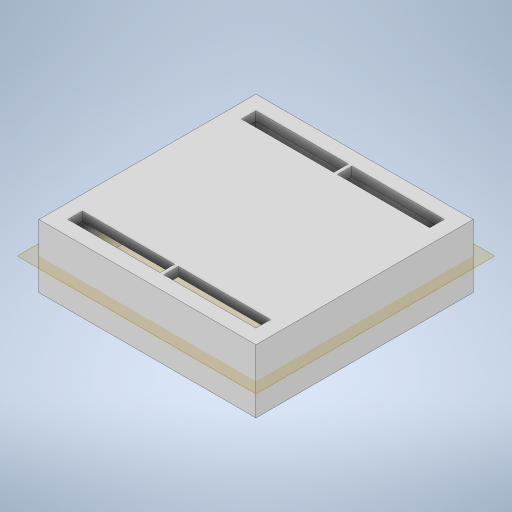
# Autodesk Inventor part: Bot v1
Saved by Autodesk Inventor 2024 (Build 280153000, 153)
## iProperties
Created: 2023-09-24
Part Number: Bot v1
Material: Generic
Document SubType Name: Modeling
Designer: CJ110
Density: 1 g/cm^3
Appearance: Default
Author: CJ110
Autodesk Inventor part; units mm, degrees
ref_plane "YZ Plane" through (0, 0, 0) normal (1, 0, 0) x (0, 1, 0)
ref_plane "XZ Plane" through (0, 0, 0) normal (0, 1, 0) x (-1, 0, 0)
ref_plane "XY Plane" through (0, 0, 0) normal (0, 0, 1) x (1, 0, 0)
sketch "Sketch1" plane through (0, 0, 0) normal (0, 1, 0) x (-1, 0, 0)
  line L0 (0, 0) -> (152.4, 0)
  line L1 (152.4, 0) -> (152.4, 152.4)
  line L2 (152.4, 152.4) -> (0, 152.4)
  line L3 (0, 152.4) -> (0, 0)
  dimension "d0" = 152.4
  dimension "d1" = 152.4
  constraints: 8 end point, 2 parallel, 1 horizontal, 1 perpendicular
  measures "d0" distance of L0.start L0.end
  measures "d1" distance of L2.end L0.start
extrude "Extrusion1" add sketch "Sketch1" along normal blind 6.35
sketch "Sketch2" plane through (0, 6.35, 0) normal (0, 1, 0) x (1, 0, 0)
  line L0 (-142.24, -142.24) -> (-77.47, -142.24)
  line L1 (-77.47, -142.24) -> (-77.47, -132.08)
  line L2 (-77.47, -132.08) -> (-142.24, -132.08)
  line L3 (-142.24, -132.08) -> (-142.24, -142.24)
  line L4 (-74.93, -142.24) -> (-10.16, -142.24)
  line L5 (-10.16, -142.24) -> (-10.16, -132.08)
  line L6 (-10.16, -132.08) -> (-74.93, -132.08)
  line L7 (-74.93, -132.08) -> (-74.93, -142.24)
  line L8 (-152.4, 0) -> (-152.4, -152.4) projected
  line L9 (-152.4, -152.4) -> (0, -152.4) projected
  line L10 (0, -152.4) -> (0, 0) projected
  line L11 (-152.4, -76.2) -> (0, -76.2) construction
  line L12 (-142.24, -10.16) -> (-77.47, -10.16)
  line L13 (-77.47, -10.16) -> (-77.47, -20.32)
  line L14 (-77.47, -20.32) -> (-142.24, -20.32)
  line L15 (-142.24, -20.32) -> (-142.24, -10.16)
  line L16 (-74.93, -10.16) -> (-10.16, -10.16)
  line L17 (-10.16, -10.16) -> (-10.16, -20.32)
  line L18 (-10.16, -20.32) -> (-74.93, -20.32)
  line L19 (-74.93, -20.32) -> (-74.93, -10.16)
  point P0 (-10.16, -137.16)
  point P1 (-10.16, -15.24)
  dimension "d4" = 10.16
  dimension "d5" = 10.16
  dimension "d6" = 10.16
  dimension "d7" = 64.77
  dimension "d8" = 64.77
  dimension "d9" = 10.16
  dimension "d10" = 10.16
  dimension "d11" = 10.16
  constraints: 34 end point, 9 symmetric about line, 4 parallel, 3 midpoint, 2 horizontal, 2 perpendicular
  measures "d4" distance between parallel lines of L8 L3
  measures "d5" distance between parallel lines of L9 L0
  measures "d6" distance between parallel lines of L0 L2
  measures "d7" distance of L0.start L0.end
  measures "d8" distance of L4.start L4.end
  measures "d9" distance from line of L10 point (-10.16, -137.16)
  measures "d10" distance between parallel lines of L9 L4
  measures "d11" distance between parallel lines of L4 L6
extrude "Extrusion2" cut sketch "Sketch2" against normal through all
sketch "Sketch3" plane through (0, 6.35, 0) normal (0, 1, 0) x (1, 0, 0)
  line L0 (-77.47, -20.32) -> (-142.24, -20.32) projected
  line L1 (-142.24, -20.32) -> (-142.24, -10.16) projected
  line L2 (-142.24, -10.16) -> (-77.47, -10.16) projected
  line L3 (-77.47, -10.16) -> (-77.47, -20.32) projected
  line L4 (-74.93, -132.08) -> (-10.16, -132.08) projected
  line L5 (-10.16, -132.08) -> (-10.16, -142.24) projected
  line L6 (-10.16, -142.24) -> (-74.93, -142.24) projected
  line L7 (-74.93, -142.24) -> (-74.93, -132.08) projected
  line L8 (-10.16, -10.16) -> (-10.16, -20.32) projected
  line L9 (-10.16, -20.32) -> (-74.93, -20.32) projected
  line L10 (-74.93, -20.32) -> (-74.93, -10.16) projected
  line L11 (-74.93, -10.16) -> (-10.16, -10.16) projected
  line L12 (-142.24, -132.08) -> (-77.47, -132.08) projected
  line L13 (-77.47, -132.08) -> (-77.47, -142.24) projected
  line L14 (-77.47, -142.24) -> (-142.24, -142.24) projected
  line L15 (-142.24, -142.24) -> (-142.24, -132.08) projected
  line L16 (-152.4, 0) -> (-152.4, -152.4) projected
  line L17 (-152.4, -152.4) -> (0, -152.4) projected
  line L18 (0, -152.4) -> (0, 0) projected
  line L19 (0, 0) -> (-152.4, 0) projected
  line L20 (-146.05, -146.05) -> (-146.05, -6.35)
  line L21 (-146.05, -6.35) -> (-6.35, -6.35)
  line L22 (-6.35, -6.35) -> (-6.35, -146.05)
  line L23 (-6.35, -146.05) -> (-146.05, -146.05)
  dimension "d14" = 6.35
  constraints: 8 end point, 3 other
  measures "d14" distance between parallel lines of L16 L20
extrude "Extrusion3" add sketch "Sketch3" along normal blind 38.1 contours L19 L18 L17 L16
ref_plane "Work Plane1" through (0, 22.225, 0) normal (0, 1, 0) x (1, 0, 0)
mirror "Mirror1" about plane through (0, 22.225, 0) normal (0, 1, 0) of "Extrusion1", "Extrusion2"
equation "\"d8\" = d7"
equation "\"d9\" = d4"
equation "\"d10\" = d5"
equation "\"d11\" = d6"
body "Solid1"
